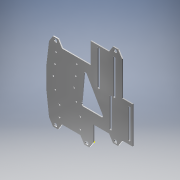
# Autodesk Inventor part: base_plate
Saved by Autodesk Inventor 2018 (Build 220112000, 112)
## iProperties
Created: 2018-04-04
Part Number: base_plate
Material: アルミニウム 6061
Document SubType Name: モデリング
Designer: NaMACHAN
Density: 2.7 g/cm^3
Appearance: アルミニウム - フラット
Sheet Metal Rule: Default
Mass: 92.2429 g
Surface Area: 369.048 cm^2
Volume: 34.164 cm^3
Author: NaMACHAN
Autodesk Inventor part; units mm, degrees
ref_plane "YZ Plane" through (0, 0, 0) normal (1, 0, 0) x (0, 1, 0)
ref_plane "XZ Plane" through (0, 0, 0) normal (0, 1, 0) x (-1, 0, 0)
ref_plane "XY Plane" through (0, 0, 0) normal (0, 0, 1) x (1, 0, 0)
sketch "スケッチ1" plane through (0, 0, 0) normal (0, 1, 0) x (-1, 0, 0)
  line L0 (85, 0) -> (90, 42)
  line L1 (90, 42) -> (90, 84)
  line L2 (90, 84) -> (85, 126)
  line L3 (-55, 101) -> (-55, 166)
  line L4 (0, 0) -> (0, 30)
  line L5 (-75, 101) -> (-55, 101)
  line L6 (5, 126) -> (5, 166)
  line L7 (-30, 166) -> (5, 166)
  line L8 (-47.5, 178) -> (-37.5, 178)
  line L9 (-37.5, 178) -> (-30, 166)
  line L10 (77.5, 138) -> (67.5, 138)
  line L11 (5, 126) -> (60, 126)
  line L12 (60, 126) -> (67.5, 138)
  line L13 (85, 126) -> (77.5, 138)
  line L14 (-47.5, 178) -> (-55, 166)
  line L15 (85, 0) -> (77.5, -12)
  line L16 (77.5, -12) -> (67.5, -12)
  line L17 (67.5, -12) -> (60, 0)
  line L18 (60, 0) -> (25, 0)
  line L19 (25, 0) -> (17.5, -12)
  line L20 (17.5, -12) -> (7.5, -12)
  line L21 (7.5, -12) -> (0, 0)
  line L22 (0, 30) -> (-30, 30)
  line L23 (-30, 30) -> (-37.5, 18)
  line L24 (-37.5, 18) -> (-47.5, 18)
  line L25 (-47.5, 18) -> (-55, 30)
  line L26 (-75, 101) -> (-75, 31)
  line L27 (-55, 30) -> (-55, 31)
  line L28 (-55, 31) -> (-75, 31)
  dimension "d219" = 20
  dimension "d222" = 10
  dimension "d224" = 10
  dimension "d227" = 7.5
  dimension "d228" = 12
  dimension "d230" = 7.5
  dimension "d231" = 12
  dimension "d233" = 10
  dimension "d234" = 10
  dimension "d235" = 7.5
  dimension "d236" = 7.5
  dimension "d238" = 7.5
  dimension "d240" = 10
  dimension "d241" = 7.5
  dimension "d242" = 12
  dimension "d275" = 65
  dimension "d276" = 7.5
  dimension "d277" = 70
  dimension "d278" = 5
  dimension "d279" = 55
  dimension "d280" = 40
  dimension "d281" = 60
  dimension "d282" = 42
  dimension "d283" = 42
  dimension "d284" = 42
  dimension "d285" = 7.5
  dimension "d286" = 12
  dimension "d287" = 7.5
  dimension "d288" = 90
  dimension "d289" = 7.5
  dimension "d290" = 30
  constraints: 58 end point, 6 horizontal, 6 horizontal alignment, 4 vertical alignment, 3 parallel, 3 perpendicular, 3 vertical, 1 coincident
  measures "d219" distance of L5.start L3.start
  measures "d222" distance of L8.start L8.end
  measures "d224" distance of L10.start L10.end
  measures "d227" horizontal distance of L10.end L11.end
  measures "d228" vertical distance of L10.start L2.end
  measures "d230" horizontal distance of L3.end L8.start
  measures "d231" vertical distance of L8.start L3.end
  measures "d233" distance of L15.end L16.end
  measures "d234" distance of L19.end L20.end
  measures "d235" horizontal distance of L0.start L15.end
  measures "d236" horizontal distance of point (0, 0) L20.end
  measures "d238" horizontal distance of L17.end L16.end
  measures "d240" distance of L23.end L24.end
  measures "d241" horizontal distance of L23.end L22.end
  measures "d242" distance from line of L25.end L24
  measures "d275" distance between parallel lines of L7 L5
  measures "d276" horizontal distance of L25.end L24.end
  measures "d277" distance of L5.start L26.end
  measures "d278" distance from line of L1 L2.end
  measures "d279" distance of L6.start L11.end
  measures "d280" distance of L6.start L6.end
  measures "d281" distance between parallel lines of L6 L3
  measures "d282" vertical distance of L2.end L1.end
  measures "d283" distance of L0.end L1.end
  measures "d284" vertical distance of L0.start L0.end
  measures "d285" horizontal distance of L18.end L19.end
  measures "d286" distance from line of L0.start L16
  measures "d287" horizontal distance of L2.end L10.start
  measures "d288" distance between parallel lines of L1 L4
  measures "d289" horizontal distance of L8.end L7.start
  measures "d290" distance of L4.start L4.end
extrude "押し出し1" add sketch "スケッチ1" along normal blind 2
fillet "フィレット1" radius 2 4 edges at (47.5, 1, 178) (-85, 1, 126) (0, 1, 0) (-85, 1, 0)
sketch "スケッチ8" plane through (0, 2, 0) normal (0, 1, 0) x (1, 0, 0)
  point P0 (0, 0)
  point P1 (-65, -9.5)
  point P2 (-25, -9.5)
  point P3 (-25, -30.5)
  point P4 (-65, -30.5)
  point P5 (-73, -51.5)
  point P6 (-33, -51.5)
  point P7 (-77, -72.5)
  point P8 (-37, -72.5)
  point P9 (-34, -93.5)
  point P10 (-74, -93.5)
  point P11 (-72, -114.5)
  point P12 (-32, -114.5)
  dimension "d132" = 40
  dimension "d133" = 40
  dimension "d134" = 40
  dimension "d135" = 40
  dimension "d136" = 40
  dimension "d137" = 40
  dimension "d138" = 9.5
  dimension "d139" = 25
  dimension "d141" = 21
  dimension "d143" = 21
  dimension "d144" = 21
  dimension "d145" = 21
  dimension "d146" = 21
  dimension "d147" = 8
  dimension "d148" = 4
  dimension "d149" = 3
  dimension "d150" = 2
  constraints: 6 horizontal alignment, 1 vertical alignment
  measures "d132" distance of point (-25, -9.5) point (-65, -9.5)
  measures "d133" distance of point (-65, -30.5) point (-25, -30.5)
  measures "d134" distance of point (-73, -51.5) point (-33, -51.5)
  measures "d135" distance of point (-77, -72.5) point (-37, -72.5)
  measures "d136" distance of point (-34, -93.5) point (-74, -93.5)
  measures "d137" distance of point (-32, -114.5) point (-72, -114.5)
  measures "d138" vertical distance of point (0, 0) point (-25, -9.5)
  measures "d139" horizontal distance of point (0, 0) point (-25, -9.5)
  measures "d141" distance of point (-25, -30.5) point (-25, -9.5)
  measures "d143" vertical distance of point (-33, -51.5) point (-25, -30.5)
  measures "d144" vertical distance of point (-37, -72.5) point (-33, -51.5)
  measures "d145" vertical distance of point (-34, -93.5) point (-37, -72.5)
  measures "d146" vertical distance of point (-32, -114.5) point (-34, -93.5)
  measures "d147" horizontal distance of point (-25, -30.5) point (-33, -51.5)
  measures "d148" horizontal distance of point (-37, -72.5) point (-33, -51.5)
  measures "d149" horizontal distance of point (-34, -93.5) point (-37, -72.5)
  measures "d150" horizontal distance of point (-34, -93.5) point (-32, -114.5)
hole "穴6" at (-65, 2, 9.5) at (-25, 2, 9.5) at (-25, 2, 30.5) at (-65, 2, 30.5) at (-73, 2, 51.5) at (-33, 2, 51.5) at (-77, 2, 72.5) at (-37, 2, 72.5) at (-34, 2, 93.5) at (-74, 2, 93.5) at (-72, 2, 114.5) at (-32, 2, 114.5) direction (0, -1, 0) diameter 3 end through all
sketch "スケッチ11" plane through (0, 2, 0) normal (0, 1, 0) x (1, 0, 0)
  line L0 (42, -96) -> (42, -161)
  arc A0 (38, -161) -> (42, -161) centre (40, -161) ccw
  line L1 (38, -161) -> (38, -96)
  arc A1 (42, -96) -> (38, -96) centre (40, -96) ccw
  line L2 (12, -96) -> (12, -161)
  arc A2 (8, -161) -> (12, -161) centre (10, -161) ccw
  line L3 (8, -161) -> (8, -96)
  arc A3 (12, -96) -> (8, -96) centre (10, -96) ccw
  line L4 (-5, -166) -> (30, -166) projected
  line L5 (-5, -126) -> (-5, -166) projected
  point P0 (0, 0)
  point P1 (50, -163)
  dimension "d194" = 2
  dimension "d198" = 2
  dimension "d199" = 30
  dimension "d220" = 5
  dimension "d221" = 70
  dimension "d256" = 15
  constraints: 8 end point, 8 point on circle, 8 tangent, 4 centre point, 2 horizontal alignment, 2 parallel, 2 vertical
  measures "d194" radius of A1
  measures "d198" radius of A2
  measures "d199" distance of A0.centre A2.centre
  measures "d220" distance from line of L4 A0.centre
  measures "d221" distance from line of A1.centre L4
  measures "d256" distance from line of L5 A2.centre
extrude "押し出し3" cut sketch "スケッチ11" against normal blind 10
sketch "スケッチ12" plane through (0, 2, 0) normal (0, 1, 0) x (1, 0, 0)
  point P0 (0, 0)
sketch "スケッチ13" plane through (0, 2, 0) normal (0, 1, 0) x (1, 0, 0)
  line L0 (67, -93) -> (67, -39)
  arc A0 (71, -39) -> (67, -39) centre (69, -39) ccw
  line L1 (71, -39) -> (71, -93)
  arc A1 (67, -93) -> (71, -93) centre (69, -93) ccw
  line L2 (29, -93) -> (29, -39)
  arc A2 (29, -39) -> (25, -39) centre (27, -39) ccw
  line L3 (25, -39) -> (25, -93)
  arc A3 (25, -93) -> (29, -93) centre (27, -93) ccw
  line L4 (55, -101) -> (75, -101) projected
  line L5 (30, -30) -> (0, -30) projected
  line L6 (75, -31) -> (55, -31) projected
  line L7 (75, -101) -> (75, -31) projected
  point P0 (0, 0)
  dimension "d205" = 2
  dimension "d206" = 2
  dimension "d208" = 8
  dimension "d210" = 42
  dimension "d291" = 8
  dimension "d292" = 6
  constraints: 8 end point, 8 point on circle, 8 tangent, 4 centre point, 2 horizontal alignment, 2 parallel, 2 vertical
  measures "d205" radius of A3
  measures "d206" radius of A1
  measures "d208" distance from line of L4 A1.centre
  measures "d210" distance of A0.centre A2.centre
  measures "d291" distance from line of L6 A0.centre
  measures "d292" distance from line of L7 A0.centre
extrude "押し出し4" cut sketch "スケッチ13" against normal blind 10
sketch "スケッチ14" plane through (0, 0, 0) normal (0, -1, 0) x (1, 0, 0)
  line L0 (-67.5, 138) -> (-77.5, 138) projected
  line L1 (-77.5, -12) -> (-67.5, -12) projected
  line L2 (-17.5, -12) -> (-7.5, -12) projected
  line L3 (37.5, 18) -> (47.5, 18) projected
  line L4 (46.3915, 178) -> (37.5, 178) projected
  point P0 (0, 0)
  point P1 (-72.5, -7)
  point P2 (-12.5, -7)
  point P3 (-72.5, 133)
  point P4 (42.5, 23)
  point P5 (41.9458, 173)
  point P6 (-72.5, 138)
  point P7 (-72.5, -12)
  point P8 (-12.5, -12)
  point P9 (42.5, 18)
  point P10 (41.9458, 178)
  dimension "d244" = 5
  dimension "d245" = 5
  dimension "d246" = 5
  dimension "d247" = 5
  dimension "d248" = 5
  constraints: 5 midpoint, 5 vertical alignment
  measures "d244" distance from line of point (41.946, 173) L4
  measures "d245" distance from line of point (-72.5, 133) L0
  measures "d246" distance from line of L1 point (-72.5, -7)
  measures "d247" distance of point (-12.5, -12) point (-12.5, -7)
  measures "d248" distance from line of L3 point (42.5, 23)
hole "穴9" at (41.9458, 0, 173) at (-72.5, 0, 133) at (-72.5, 0, -7) at (-12.5, 0, -7) at (42.5, 0, 23) direction (0, 1, 0) diameter 6 end through all
sketch "スケッチ16" plane through (0, 2, 0) normal (0, 1, 0) x (1, 0, 0)
  line L0 (-12.0118, -106.2661) -> (17.8753, -54.5)
  arc A0 (17.8753, -54.5) -> (15.2773, -50) centre (15.2773, -53) ccw
  line L1 (15.2773, -50) -> (-20, -50)
  arc A1 (-20, -50) -> (-22.5981, -54.5) centre (-20, -53) ccw
  line L2 (-22.5981, -54.5) -> (-17.9882, -106.2661)
  arc A2 (-17.9882, -106.2661) -> (-12.0118, -106.2661) centre (-15, -106) ccw
  line L3 (30, -30) -> (0, -30) projected
  line L4 (-60, -126) -> (-5, -126) projected
  point P0 (0, 0)
  dimension "d264" = 20
  dimension "d265" = 20
  dimension "d266" = 20
  dimension "d267" = 3
  dimension "d268" = 3
  dimension "d269" = 3
  dimension "d270" = 120
  dimension "d271" = 120
  dimension "d272" = 10
  constraints: 6 end point, 6 point on circle, 4 tangent, 3 centre point, 1 horizontal, 1 horizontal alignment
  measures "d264" distance between parallel lines of L3 L1
  measures "d265" distance from line of L4 A2.centre
  measures "d266" horizontal distance of A1.centre L3.end
  measures "d267" radius of A1
  measures "d268" radius of A0
  measures "d269" radius of A2
  measures "d272" horizontal distance of L4.end A2.centre
extrude "押し出し6" cut sketch "スケッチ16" against normal blind 10
